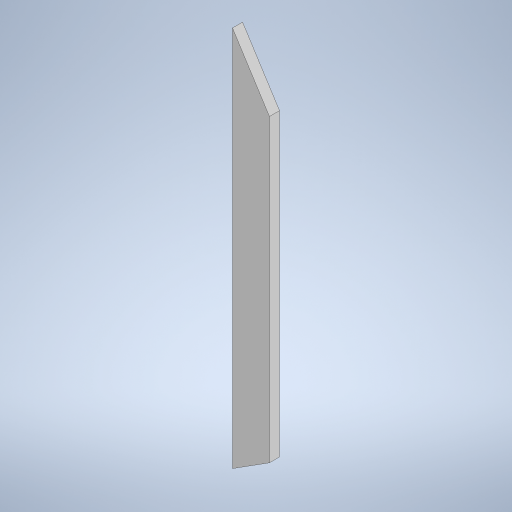
# Autodesk Inventor part: angled triangle beam
Saved by Autodesk Inventor 2023 (Build 270158000, 158)
## iProperties
Created: 2022-08-19
Part Number: angled triangle beam
Material: Generic
Document SubType Name: Modeling
Designer: rkant
Density: 1 g/cm^3
Appearance: Default
Author: rkant
Autodesk Inventor part; units mm, degrees
ref_plane "YZ Plane" through (0, 0, 0) normal (1, 0, 0) x (0, 1, 0)
ref_plane "XZ Plane" through (0, 0, 0) normal (0, 1, 0) x (-1, 0, 0)
ref_plane "XY Plane" through (0, 0, 0) normal (0, 0, 1) x (1, 0, 0)
sketch "Sketch1" plane through (0, 0, 0) normal (1, 0, 0) x (0, 1, 0)
  line L0 (-721.6775, 19.05) -> (721.6775, 19.05)
  line L1 (721.6775, 19.05) -> (721.6775, -19.05)
  line L2 (721.6775, -19.05) -> (-721.6775, -19.05)
  line L3 (-721.6775, -19.05) -> (-721.6775, 19.05)
  line L4 (-721.6775, 19.05) -> (721.6775, -19.05) construction
  line L5 (721.6775, 19.05) -> (-721.6775, -19.05) construction
  point P0 (0, 0)
  dimension "d0" = 38.1
  dimension "d1" = 1443.355
  constraints: 12 end point, 2 midpoint, 2 parallel, 1 horizontal, 1 perpendicular
  measures "d0" distance of L0.end L1.end
  measures "d1" distance of L1.end L2.end
extrude "Extrusion1" add sketch "Sketch1" along normal blind 139.7
sketch "Sketch2" plane through (0, -721.6775, 19.05) normal (0, 0, 1) x (1, 0, 0)
  line L0 (0, 0) -> (0, 1443.355) projected
  line L1 (0, 1443.355) -> (139.7, 1223.223)
  line L2 (139.7, 0) -> (139.7, 1443.355) projected
  line L3 (0, 1443.355) -> (139.7, 1443.355) projected
  line L4 (0, 0) -> (139.7, 88.6563)
  line L5 (0, 0) -> (139.7, 0) projected
  point P0 (0, 721.6775)
  dimension "d4" = 57.6
  dimension "d5" = 32.4
  constraints: 4 end point, 2 point on line
  measures "d4" angle of L3 L1
  measures "d5" angle of L5 L4
extrude "Extrusion2" cut sketch "Sketch2" against normal blind 38.1 contours L4 L2 L5 | L3 L2 L1
body "Solid1"
